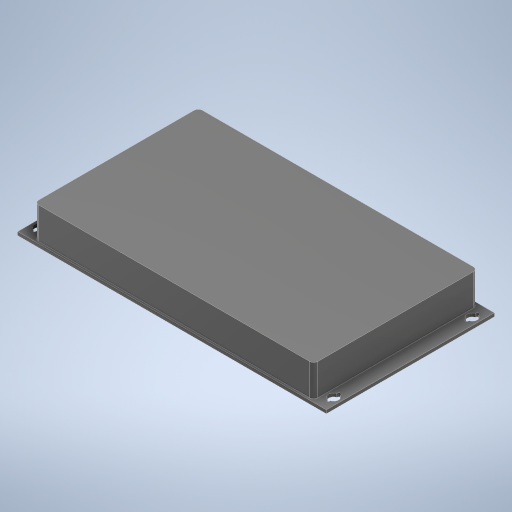
# Autodesk Inventor part: SUSTAINA-POWER-MONITOR-BOARD
Saved by Autodesk Inventor 2024.2 (Build 282272000, 272)
## iProperties
Created: 2024-01-24
Part Number: SUSTAINA-POWER-MONITOR-BOARD
Material: Acetal Resin, Black
Document SubType Name: Modeling
Designer: Masato Kubotera
Density: 1.425 g/cm^3
Appearance: Smooth - Black
Mass: 115.124 g
Surface Area: 165.657 cm^2
Volume: 80.7888 cm^3
Author: Masato Kubotera
Autodesk Inventor part; units mm, degrees
ref_plane "YZ Plane" through (0, 0, 0) normal (1, 0, 0) x (0, 1, 0)
ref_plane "XZ Plane" through (0, 0, 0) normal (0, 1, 0) x (-1, 0, 0)
ref_plane "XY Plane" through (0, 0, 0) normal (0, 0, 1) x (1, 0, 0)
sketch "Sketch1" plane through (0, 0, 0) normal (0, 0, 1) x (1, 0, 0)
  line L0 (40, 73.5) -> (-40, 73.5)
  line L1 (-40, 73.5) -> (-40, -73.5)
  line L2 (-40, -73.5) -> (40, -73.5)
  line L3 (40, -73.5) -> (40, 73.5)
  line L4 (40, 73.5) -> (-40, -73.5) construction
  line L5 (-40, 73.5) -> (40, -73.5) construction
  line L6 (-33, 70) -> (33, 70) construction
  line L7 (33, 70) -> (33, -70) construction
  line L8 (33, -70) -> (-33, -70) construction
  line L9 (-33, -70) -> (-33, 70) construction
  line L10 (-33, 70) -> (33, -70) construction
  line L11 (33, 70) -> (-33, -70) construction
  line L12 (40, 0) -> (-40, 0) construction
  line L13 (0, 73.5) -> (0, -73.5) construction
  circle A0 centre (33, 70) radius 2.4
  circle A1 centre (-33, 70) radius 2.4
  circle A2 centre (33, -70) radius 2.4
  circle A3 centre (-33, -70) radius 2.4
  line L14 (33, 73.25) -> (33, 66.75) construction
  arc A4 (35.2895, 69.2801) -> (35.2895, 70.7199) centre (35.5, 70) ccw
  arc A5 (30.7105, 70.7199) -> (30.7105, 69.2801) centre (30.5, 70) ccw
  arc A6 (-35.2895, 70.7199) -> (-35.2895, 69.2801) centre (-35.5, 70) ccw
  arc A7 (-30.7105, 69.2801) -> (-30.7105, 70.7199) centre (-30.5, 70) ccw
  arc A8 (35.2895, -70.7199) -> (35.2895, -69.2801) centre (35.5, -70) ccw
  arc A9 (30.7105, -69.2801) -> (30.7105, -70.7199) centre (30.5, -70) ccw
  arc A10 (-35.2895, -69.2801) -> (-35.2895, -70.7199) centre (-35.5, -70) ccw
  arc A11 (-30.7105, -70.7199) -> (-30.7105, -69.2801) centre (-30.5, -70) ccw
  line L15 (39, 66.5) -> (-39, 66.5)
  line L16 (-39, 66.5) -> (-39, -66.5)
  line L17 (-39, -66.5) -> (39, -66.5)
  line L18 (39, -66.5) -> (39, 66.5)
  line L19 (39, 66.5) -> (-39, -66.5) construction
  line L20 (-39, 66.5) -> (39, -66.5) construction
  point P0 (0, 0)
  point P1 (36.25, 70)
  point P2 (29.75, 70)
  point P3 (36.25, -70)
  point P4 (30.7105, 69.2801)
  point P5 (30.7105, 70.7199)
  point P6 (-30.7105, 70.7199)
  point P7 (-30.7105, 69.2801)
  point P8 (-35.2895, 69.2801)
  point P9 (-35.2895, 70.7199)
  point P10 (-30.7105, -69.2801)
  point P11 (-30.7105, -70.7199)
  point P12 (-35.2895, -70.7199)
  point P13 (-35.2895, -69.2801)
  point P14 (35.2895, -69.2801)
  point P15 (35.2895, -70.7199)
  point P16 (30.7105, -70.7199)
  point P17 (30.7105, -69.2801)
  dimension "d0" = 80
  dimension "d1" = 147
  dimension "d19" = 4.8
  dimension "d30" = 6.5
  dimension "d33" = 140
  dimension "d34" = 66
  dimension "d35" = 6.5
  dimension "d36" = 1.5
  dimension "d37" = 7
  dimension "d38" = 1
  dimension "d39" = 133
  dimension "d40" = 78
  dimension "d41" = 14
  constraints: 42 end point, 25 symmetric about line, 20 point on circle, 12 centre point, 11 midpoint, 6 coincident, 6 parallel, 3 horizontal, 3 perpendicular, 1 point on line, 1 vertical, 11 other
  measures "d0" distance of L2.end L1.end
  measures "d1" distance of L1.end L0.end
  measures "d19" diameter of A0
  measures "d30" distance of L14.start L14.end
  measures "d33" distance of L8.end L6.start
  measures "d34" distance of L7.end L8.end
  measures "d35" distance of point (36.25, 70) point (29.75, 70)
  measures "d36" diameter of A4
  measures "d37" diameter of L0 L6
  measures "d38" distance between parallel lines of L3 L18
  measures "d39" distance of L15.end L16.end
  measures "d40" distance of L15.start L15.end
  measures "d41" diameter of L3 L7
extrude "Extrusion1" add sketch "Sketch1" along normal blind 1.6 contours L3 L2 L1 L0 | L18 L17 L16 L15
extrude "Extrusion2" add sketch "Sketch1" along normal blind 16.6 contours L18 L17 L16 L15
fillet "Fillet1" radius 2 4 edges at (39, -66.5, 9.1) (39, 66.5, 9.1) (-39, -66.5, 9.1) (-39, 66.5, 9.1)
body "Solid1"
